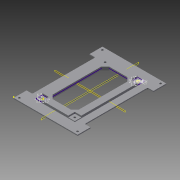
# Autodesk Inventor part: transillum_diffusor_partE_v1
Saved by Autodesk Inventor 2015 (Build 190159000, 159)
## iProperties
Created: 2022-05-26
Part Number: transillum_diffusor_partE_v1
Material: Genérico
Document SubType Name: Modeling
Designer: Zuloaga
Density: 1 g/cm^3
Appearance: Valor por defecto
Author: Zuloaga
Autodesk Inventor part; units mm, degrees
ref_plane "YZ Plane" through (0, 0, 0) normal (1, 0, 0) x (0, 1, 0)
ref_plane "XZ Plane" through (0, 0, 0) normal (0, 1, 0) x (-1, 0, 0)
ref_plane "XY Plane" through (0, 0, 0) normal (0, 0, 1) x (1, 0, 0)
sketch "Boceto1" plane through (0, 0, 0) normal (0, 0, 1) x (1, 0, 0)
  line L0 (0, 0) -> (127.5, 0)
  line L1 (127.5, 0) -> (127.5, 177)
  line L2 (127.5, 177) -> (0, 177)
  line L3 (0, 177) -> (0, 0)
  dimension "d32" = 127.5
  dimension "d33" = 177
  constraints: 8 end point, 2 parallel, 1 horizontal, 1 perpendicular
  measures "d32" distance of L2.end L1.end
  measures "d33" distance of L1.end L0.end
extrude "Extrusión1" add sketch "Boceto1" along normal blind 6
ref_plane "Plano de trabajo6" through (0, 88.5, 0) normal (0, -1, 0) x (1, 0, 0)
ref_plane "Plano de trabajo7" through (63.75, 0, 0) normal (-1, 0, 0) x (0, 0, 1)
sketch "Boceto17" plane through (0, 0, 6) normal (0, 0, 1) x (1, 0, 0)
  line L0 (127.5, 0) -> (116, 0)
  line L1 (116, 0) -> (116, 11.5)
  line L2 (116, 11.5) -> (127.5, 11.5)
  line L3 (127.5, 11.5) -> (127.5, 0)
  line L4 (0, 0) -> (11.5, 0)
  line L5 (11.5, 0) -> (11.5, 11.5)
  line L6 (11.5, 11.5) -> (0, 11.5)
  line L7 (0, 11.5) -> (0, 0)
  line L8 (127.5, 177) -> (116, 177)
  line L9 (116, 177) -> (116, 165.5)
  line L10 (116, 165.5) -> (127.5, 165.5)
  line L11 (127.5, 165.5) -> (127.5, 177)
  line L12 (0, 177) -> (11.5, 177)
  line L13 (11.5, 177) -> (11.5, 165.5)
  line L14 (11.5, 165.5) -> (0, 165.5)
  line L15 (0, 165.5) -> (0, 177)
  dimension "d124" = 11.5
  dimension "d125" = 11.5
  dimension "d129" = 11.5
  dimension "d130" = 11.5
  dimension "d131" = 11.5
  dimension "d132" = 11.5
  dimension "d133" = 11.5
  dimension "d134" = 11.5
  constraints: 32 end point, 8 parallel, 4 horizontal, 4 perpendicular
  measures "d124" distance of L1.end L2.end
  measures "d125" distance of L0.end L1.end
  measures "d129" distance of L6.end L5.end
  measures "d130" distance of L5.end L4.end
  measures "d131" distance of L10.end L9.end
  measures "d132" distance of L9.end L8.end
  measures "d133" distance of L13.end L14.end
  measures "d134" distance of L12.end L13.end
extrude "Extrusión12" cut sketch "Boceto17" against normal blind 4
sketch "Boceto18" plane through (0, 0, 2) normal (0, 0, 1) x (1, 0, 0)
  line L0 (0, 0) -> (11.5, 0)
  line L1 (11.5, 0) -> (11.5, 11.5)
  line L2 (11.5, 11.5) -> (0, 11.5)
  line L3 (0, 11.5) -> (0, 0)
  line L4 (127.5, 0) -> (116, 0)
  line L5 (116, 0) -> (116, 11.5)
  line L6 (116, 11.5) -> (127.5, 11.5)
  line L7 (127.5, 11.5) -> (127.5, 0)
  line L8 (127.5, 177) -> (116, 177)
  line L9 (116, 177) -> (116, 165.5)
  line L10 (116, 165.5) -> (127.5, 165.5)
  line L11 (127.5, 165.5) -> (127.5, 177)
  line L12 (0, 177) -> (11.5, 177)
  line L13 (11.5, 177) -> (11.5, 165.5)
  line L14 (11.5, 165.5) -> (0, 165.5)
  line L15 (0, 165.5) -> (0, 177)
  line L16 (116, 11.5) -> (127.5, 0)
  line L17 (127.5, 11.5) -> (116, 0)
  circle A0 centre (121.75, 5.75) radius 2
  dimension "d137" = 4
  constraints: 36 end point, 8 parallel, 5 perpendicular, 4 horizontal, 2 point on line, 1 centre point, 1 midpoint
  measures "d137" diameter of A0
extrude "Extrusión13" cut sketch "Boceto18" against normal blind 3.2 contours A0 L17 L16 | L16 L17 A0 | A0 L16 L17 | L17 L16 A0
mirror "Simetría7" about plane through (63.75, 0, 0) normal (-1, 0, 0) of "Extrusión13"
mirror "Simetría8" about plane through (0, 88.5, 0) normal (0, -1, 0) of "Extrusión13", "Simetría7"
sketch "Boceto19" plane through (0, 0, 6) normal (0, 0, 1) x (1, 0, 0)
  line L0 (0, 0) -> (127.5, 0)
  line L1 (127.5, 0) -> (127.5, 85.5)
  line L2 (127.5, 85.5) -> (0, 85.5)
  line L3 (0, 85.5) -> (0, 0)
  line L4 (127.5, 0) -> (127.5, 177) projected
  line L5 (0, 85.5) -> (127.5, 85.5)
  line L6 (127.5, 85.5) -> (127.5, 91.5)
  line L7 (127.5, 91.5) -> (0, 91.5)
  line L8 (0, 91.5) -> (0, 85.5)
  line L9 (0, 91.5) -> (127.5, 91.5)
  line L10 (127.5, 91.5) -> (127.5, 177)
  line L11 (127.5, 177) -> (0, 177)
  line L12 (0, 177) -> (0, 91.5)
  dimension "d140" = 127.5
  dimension "d141" = 85.5
  dimension "d142" = 6
  constraints: 24 end point, 6 parallel, 3 horizontal, 3 perpendicular, 1 point on line
  measures "d140" distance of L2.end L1.end
  measures "d141" distance of L1.end L0.end
  measures "d142" distance of L6.end L5.end
extrude "Extrusión14" cut sketch "Boceto19" against normal blind 2.5
sketch "Boceto20" plane through (0, 0, 0) normal (0, 0, -1) x (-1, 0, 0)
  line L0 (-127.5, 165.5) -> (-127.5, 11.5) projected
  line L1 (-127.5, 88.5) -> (-127.5, 9.25)
  line L2 (-127.5, 0) -> (-127.5, 177) projected
  line L3 (-127.5, 88.5) -> (-48.25, 88.5) construction
  line L4 (-11.5, 0) -> (-116, 0) projected
  line L5 (-63.75, 0) -> (-102.75, 0)
  line L6 (-63.75, 0) -> (-24.75, 0) construction
  line L7 (-102.75, 0) -> (-102.75, 9.25)
  line L8 (-127.5, 9.25) -> (-102.75, 9.25)
  line L9 (-102.75, 9.25) -> (-24.75, 9.25)
  line L10 (-24.75, 9.25) -> (-24.75, 167.75)
  line L11 (-24.75, 167.75) -> (-102.75, 167.75)
  line L12 (-102.75, 167.75) -> (-102.75, 9.25)
  line L13 (-102.75, 9.25) -> (-102.75, 25.75)
  line L14 (-102.75, 25.75) -> (-96.25, 25.75)
  circle A0 centre (-96.25, 25.75) radius 2
  point P0 (0, 0)
  point P1 (-127.5, 91.5)
  point P2 (-127.5, 85.5)
  dimension "d145" = 79.25
  dimension "d146" = 90
  dimension "d149" = 39
  dimension "d150" = 180
  dimension "d151" = 78
  dimension "d152" = 158.5
  dimension "d153" = 16.5
  dimension "d154" = 6.5
  dimension "d155" = 4
  constraints: 24 end point, 4 horizontal, 2 collinear, 2 equal length, 2 midpoint, 2 parallel, 2 perpendicular, 1 centre point, 1 coincident, 1 point on line, 1 vertical
  measures "d145" distance of L1.start L1.end
  measures "d146" angle of L1 L3
  measures "d149" distance of L5.start L5.end
  measures "d150" angle of L5 L6
  measures "d151" distance of L11.end L10.end
  measures "d152" distance of L10.end L9.end
  measures "d153" distance of L7.end L13.end
  measures "d154" distance of L13.end L14.end
  measures "d155" diameter of A0
extrude "Extrusión15" cut sketch "Boceto20" against normal blind 10 contours A0
mirror "Simetría9" about plane through (0, 88.5, 0) normal (0, -1, 0) of "Extrusión15"
mirror "Simetría10" about plane through (63.75, 0, 0) normal (-1, 0, 0) of "Extrusión15", "Simetría9"
sketch "Boceto21" plane through (0, 0, 3.5) normal (0, 0, 1) x (1, 0, 0)
  circle A0 centre (31.25, 25.75) radius 2 projected
  line L0 (31.25, 25.75) -> (24.75, 25.75)
  line L1 (24.75, 25.75) -> (24.75, 32.25)
  line L2 (24.75, 32.25) -> (37.75, 32.25)
  line L3 (37.75, 32.25) -> (37.75, 19.25)
  line L4 (37.75, 19.25) -> (24.75, 19.25)
  line L5 (24.75, 19.25) -> (24.75, 32.25)
  circle A1 centre (96.25, 151.25) radius 2 projected
  line L6 (96.25, 151.25) -> (102.75, 151.25)
  line L7 (96.25, 151.25) -> (102.75, 151.25) construction
  line L8 (102.75, 151.25) -> (102.75, 157.75)
  line L9 (102.75, 157.75) -> (89.75, 157.75)
  line L10 (89.75, 157.75) -> (89.75, 144.75)
  line L11 (89.75, 144.75) -> (102.75, 144.75)
  line L12 (102.75, 144.75) -> (102.75, 157.75)
  line L13 (37.75, 32.25) -> (89.75, 32.25)
  line L14 (89.75, 32.25) -> (89.75, 144.75)
  line L15 (89.75, 144.75) -> (37.75, 144.75)
  line L16 (37.75, 144.75) -> (37.75, 32.25)
  point P0 (0, 0)
  dimension "d158" = 6.5
  dimension "d159" = 6.5
  dimension "d160" = 13
  dimension "d161" = 13
  dimension "d162" = 6.5
  dimension "d163" = 0
  dimension "d164" = 6.5
  dimension "d165" = 90
  dimension "d166" = 13
  dimension "d167" = 13
  constraints: 34 end point, 6 horizontal, 6 parallel, 5 perpendicular, 1 collinear
  measures "d158" distance of L0.start L0.end
  measures "d159" distance of L0.end L1.end
  measures "d160" distance of L3.end L4.end
  measures "d161" distance of L2.end L3.end
  measures "d162" distance of L6.start L6.end
  measures "d163" distance between parallel lines of L6 L7
  measures "d164" distance of L6.end L8.end
  measures "d165" angle of L8 L6
  measures "d166" distance of L11.end L10.end
  measures "d167" distance of L10.end L9.end
extrude "Extrusión16" cut sketch "Boceto21" against normal blind 10 contours L16 L15 L14 L13
sketch "Boceto22" plane through (0, 0, 3.5) normal (0, 0, 1) x (1, 0, 0)
  line L0 (0, 165.5) -> (11.5, 165.5)
  line L1 (0, 165.5) -> (11.5, 165.5) projected
  line L2 (11.5, 165.5) -> (11.5, 177)
  line L3 (11.5, 165.5) -> (11.5, 177) projected
  line L4 (11.5, 177) -> (116, 177)
  line L5 (116, 177) -> (116, 165.5) projected
  line L6 (116, 177) -> (116, 165.5)
  line L7 (116, 165.5) -> (127.5, 165.5)
  line L8 (116, 165.5) -> (127.5, 165.5) projected
  line L9 (127.5, 165.5) -> (127.5, 11.5)
  line L10 (127.5, 165.5) -> (127.5, 11.5) projected
  line L11 (127.5, 11.5) -> (116, 11.5)
  line L12 (127.5, 11.5) -> (116, 11.5) projected
  line L13 (116, 11.5) -> (116, 0)
  line L14 (116, 11.5) -> (116, 0) projected
  line L15 (116, 0) -> (11.5, 0)
  line L16 (11.5, 0) -> (11.5, 11.5)
  line L17 (11.5, 0) -> (11.5, 11.5) projected
  line L18 (11.5, 11.5) -> (0, 11.5)
  line L19 (11.5, 11.5) -> (0, 11.5) projected
  line L20 (0, 11.5) -> (0, 165.5)
  line L21 (37.75, 144.75) -> (89.75, 144.75)
  line L22 (89.75, 144.75) -> (89.75, 32.25)
  line L23 (89.75, 32.25) -> (37.75, 32.25)
  line L24 (37.75, 32.25) -> (37.75, 144.75)
  circle A0 centre (31.25, 25.75) radius 2
  line L25 (31.25, 25.75) -> (24.75, 25.75)
  line L26 (24.75, 25.75) -> (24.75, 32.25)
  line L27 (24.75, 32.25) -> (37.75, 32.25)
  line L28 (37.75, 32.25) -> (37.75, 19.25)
  line L29 (37.75, 19.25) -> (24.75, 19.25)
  line L30 (24.75, 19.25) -> (24.75, 32.25)
  circle A1 centre (96.25, 151.25) radius 2
  line L31 (96.25, 151.25) -> (102.75, 151.25)
  line L32 (96.25, 151.25) -> (102.75, 151.25) construction
  line L33 (102.75, 151.25) -> (102.75, 157.75)
  line L34 (102.75, 157.75) -> (89.75, 157.75)
  line L35 (89.75, 157.75) -> (89.75, 144.75)
  line L36 (89.75, 144.75) -> (102.75, 144.75)
  line L37 (102.75, 144.75) -> (102.75, 157.75)
  line L38 (37.75, 32.25) -> (89.75, 32.25)
  line L39 (89.75, 32.25) -> (89.75, 144.75)
  line L40 (89.75, 144.75) -> (37.75, 144.75)
  line L41 (37.75, 144.75) -> (37.75, 32.25)
  line L42 (24.75, 19.25) -> (102.75, 19.25)
  line L43 (102.75, 19.25) -> (102.75, 157.75)
  line L44 (102.75, 157.75) -> (24.75, 157.75)
  line L45 (24.75, 157.75) -> (24.75, 19.25)
  point P0 (0, 0)
  point P1 (0, 0)
  dimension "d170" = 6.5
  dimension "d171" = 6.5
  dimension "d172" = 13
  dimension "d173" = 13
  dimension "d174" = 6.5
  dimension "d175" = 0
  dimension "d176" = 6.5
  dimension "d177" = 90
  dimension "d178" = 13
  dimension "d179" = 13
  constraints: 74 end point, 19 equal length, 10 perpendicular, 8 horizontal, 2 centre point, 1 collinear
  measures "d170" distance of L25.start L25.end
  measures "d171" distance of L25.end L26.end
  measures "d172" distance of L28.end L29.end
  measures "d173" distance of L27.end L28.end
  measures "d174" distance of L31.start L31.end
  measures "d175" distance between parallel lines of L31 L32
  measures "d176" distance of L31.end L33.end
  measures "d177" angle of L33 L31
  measures "d178" distance of L36.end L35.end
  measures "d179" distance of L35.end L34.end
extrude "Extrusión17" cut sketch "Boceto22" against normal blind 1.5 contours L0 L2 L4 L5 L7 L9 L11 L13 L15 L16 L18 L20
sketch "Boceto23" plane through (0, 0, 2) normal (0, 0, 1) x (1, 0, 0)
  line L0 (0, 0) -> (11.5, 0)
  line L1 (11.5, 0) -> (11.5, 11.5)
  line L2 (11.5, 11.5) -> (0, 11.5)
  line L3 (0, 11.5) -> (0, 0)
  line L4 (127.5, 177) -> (116, 177)
  line L5 (116, 177) -> (116, 165.5)
  line L6 (116, 165.5) -> (127.5, 165.5)
  line L7 (127.5, 165.5) -> (127.5, 177)
  line L8 (11.5, 11.5) -> (116, 11.5)
  line L9 (116, 11.5) -> (116, 165.5)
  line L10 (116, 165.5) -> (11.5, 165.5)
  line L11 (11.5, 165.5) -> (11.5, 11.5)
  line L12 (24.75, 157.75) -> (102.75, 157.75)
  line L13 (102.75, 157.75) -> (102.75, 19.25)
  line L14 (102.75, 19.25) -> (24.75, 19.25)
  line L15 (24.75, 19.25) -> (24.75, 157.75)
  circle A0 centre (31.25, 151.25) radius 2 projected
  line L16 (31.25, 151.25) -> (0, 151.25)
  line L17 (0, 177) -> (0, 0) projected
  circle A1 centre (96.25, 25.75) radius 2 projected
  line L18 (0, 151.25) -> (11.5, 151.25)
  line L19 (11.5, 151.25) -> (11.5, 25.75)
  line L20 (11.5, 25.75) -> (0, 25.75)
  line L21 (0, 25.75) -> (0, 151.25)
  line L22 (96.25, 25.75) -> (127.5, 25.75)
  line L23 (127.5, 25.75) -> (116, 25.75)
  line L24 (116, 25.75) -> (116, 151.25)
  line L25 (116, 151.25) -> (127.5, 151.25)
  line L26 (127.5, 151.25) -> (127.5, 25.75)
  dimension "d182" = 11.5
  dimension "d183" = 11.5
  dimension "d184" = 11.5
  dimension "d185" = 11.5
  constraints: 52 end point, 12 parallel, 8 horizontal, 6 perpendicular, 3 point on line
  measures "d182" distance of L2.end L1.end
  measures "d183" distance of L1.end L0.end
  measures "d184" distance of L6.end L5.end
  measures "d185" distance of L5.end L4.end
extrude "Extrusión18" cut sketch "Boceto23" against normal blind 3 contours L17 L16 L11 L20 | L9 L25 L26 L22
fillet "Empalme1" radius 2 4 edges at (11.5, 151.25, 1) (116, 151.25, 1) (116, 25.75, 1) (11.5, 25.75, 1)
sketch "Boceto24" plane through (0, 0, 3.5) normal (0, 0, 1) x (1, 0, 0)
  line L0 (24.75, 157.75) -> (102.75, 157.75)
  line L1 (102.75, 157.75) -> (102.75, 19.25)
  line L2 (102.75, 19.25) -> (24.75, 19.25)
  line L3 (24.75, 19.25) -> (24.75, 157.75)
  circle A0 centre (31.25, 151.25) radius 2 projected
  circle A1 centre (31.25, 151.25) radius 2
  circle A2 centre (96.25, 151.25) radius 2 projected
  circle A3 centre (96.25, 151.25) radius 2
  circle A4 centre (96.25, 25.75) radius 2 projected
  circle A5 centre (96.25, 25.75) radius 2
  circle A6 centre (31.25, 25.75) radius 2 projected
  circle A7 centre (31.25, 25.75) radius 2
  line L4 (37.75, 144.75) -> (89.75, 144.75)
  line L5 (89.75, 144.75) -> (89.75, 32.25)
  line L6 (89.75, 32.25) -> (37.75, 32.25)
  line L7 (37.75, 32.25) -> (37.75, 144.75)
  point P0 (0, 0)
  constraints: 16 end point, 4 centre point, 4 coincident, 4 parallel, 2 horizontal, 2 perpendicular
extrude "Extrusión19" add sketch "Boceto24" along normal blind 3
sketch "Boceto25" plane through (0, 0, 6.5) normal (0, 0, 1) x (1, 0, 0)
  line L0 (37.75, 144.75) -> (24.75, 144.75)
  line L1 (24.75, 144.75) -> (24.75, 157.75)
  line L2 (24.75, 157.75) -> (37.75, 157.75)
  line L3 (37.75, 157.75) -> (37.75, 144.75)
  line L4 (24.75, 19.25) -> (37.75, 19.25)
  line L5 (37.75, 19.25) -> (37.75, 32.25)
  line L6 (37.75, 32.25) -> (24.75, 32.25)
  line L7 (24.75, 32.25) -> (24.75, 19.25)
  line L8 (102.75, 19.25) -> (89.75, 19.25)
  line L9 (89.75, 19.25) -> (89.75, 32.25)
  line L10 (89.75, 32.25) -> (102.75, 32.25)
  line L11 (102.75, 32.25) -> (102.75, 19.25)
  line L12 (102.75, 157.75) -> (89.75, 157.75)
  line L13 (89.75, 157.75) -> (89.75, 144.75)
  line L14 (89.75, 144.75) -> (102.75, 144.75)
  line L15 (102.75, 144.75) -> (102.75, 157.75)
  circle A0 centre (31.25, 151.25) radius 2 projected
  circle A1 centre (31.25, 151.25) radius 2
  circle A2 centre (96.25, 151.25) radius 2 projected
  circle A3 centre (96.25, 151.25) radius 2
  circle A4 centre (96.25, 25.75) radius 2 projected
  circle A5 centre (96.25, 25.75) radius 2
  circle A6 centre (31.25, 25.75) radius 2 projected
  circle A7 centre (31.25, 25.75) radius 2
  point P0 (0, 0)
  dimension "d191" = 13
  dimension "d192" = 13
  constraints: 32 end point, 8 parallel, 4 centre point, 4 coincident, 4 horizontal, 4 perpendicular, 2 point on line
  measures "d191" distance of L1.end L2.end
  measures "d192" distance of L0.end L1.end
sketch "Boceto26" plane through (0, 0, 6.5) normal (0, 0, 1) x (1, 0, 0)
  line L0 (37.75, 32.25) -> (45.75, 32.25)
  line L1 (45.75, 32.25) -> (45.75, 40.25)
  line L2 (45.75, 40.25) -> (37.75, 40.25)
  line L3 (37.75, 40.25) -> (37.75, 32.25)
  line L4 (37.75, 40.25) -> (45.75, 32.25)
  line L5 (89.75, 32.25) -> (81.75, 32.25)
  line L6 (81.75, 32.25) -> (81.75, 40.25)
  line L7 (81.75, 40.25) -> (89.75, 40.25)
  line L8 (89.75, 40.25) -> (89.75, 32.25)
  line L9 (89.75, 40.25) -> (81.75, 32.25)
  line L10 (37.75, 144.75) -> (45.75, 144.75)
  line L11 (45.75, 144.75) -> (45.75, 136.75)
  line L12 (45.75, 136.75) -> (37.75, 136.75)
  line L13 (37.75, 136.75) -> (37.75, 144.75)
  line L14 (45.75, 144.75) -> (37.75, 136.75)
  line L15 (89.75, 144.75) -> (81.75, 144.75)
  line L16 (81.75, 144.75) -> (81.75, 136.75)
  line L17 (81.75, 136.75) -> (89.75, 136.75)
  line L18 (89.75, 136.75) -> (89.75, 144.75)
  line L19 (89.75, 136.75) -> (81.75, 144.75)
  point P0 (0, 0)
  dimension "d193" = 8
  dimension "d194" = 8
  dimension "d195" = 8
  dimension "d196" = 8
  dimension "d197" = 8
  dimension "d198" = 8
  dimension "d199" = 8
  dimension "d200" = 8
  constraints: 40 end point, 8 parallel, 4 horizontal, 4 perpendicular
  measures "d193" distance of L2.end L1.end
  measures "d194" distance of L1.end L0.end
  measures "d195" distance of L6.end L7.end
  measures "d196" distance of L5.end L6.end
  measures "d197" distance of L11.end L12.end
  measures "d198" distance of L10.end L11.end
  measures "d199" distance of L17.end L16.end
  measures "d200" distance of L16.end L15.end
extrude "Extrusión20" add sketch "Boceto26" against normal blind 6.5 contours L3 L4 L0 | L5 L9 L8 | L10 L14 L13 | L18 L19 L15
extrude "Extrusión21" cut sketch "Boceto25" against normal blind 3
fillet "Empalme2" radius 1 4 edges at (89.75, 32.25, 5) (37.75, 32.25, 5) (37.75, 144.75, 5) (89.75, 144.75, 5)
